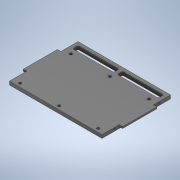
# Autodesk Inventor part: Cockpit_circuit_board_frame
Saved by Autodesk Inventor 2020.4 (Build 244396000, 396)
## iProperties
Created: 2022-01-28
Part Number: Cockpit_circuit_board_frame
Material: アセタール樹脂、黒
Document SubType Name: Modeling
Designer: Masato Kubotera
Density: 1.425 g/cm^3
Appearance: 滑らか - 黒
Author: Masato Kubotera
Autodesk Inventor part; units mm, degrees
ref_plane "YZ Plane" through (0, 0, 0) normal (1, 0, 0) x (0, 1, 0)
derived "Cockpit_side_frame.ipt"
sketch "スケッチ2" plane through (0, 0, 0) normal (0, 1, 0) x (-1, 0, 0)
  line L0 (-28.5, -22.5) -> (86.5, -22.5) construction
  line L1 (86.5, -22.5) -> (86.5, -138.5)
  line L2 (86.5, -96) -> (-28.5, -96) construction
  line L3 (-28.5, -96) -> (-28.5, -22.5) construction
  line L4 (-28.5, -22.5) -> (86.5, -96) construction
  line L5 (86.5, -22.5) -> (-28.5, -96) construction
  line L6 (36.5, -101) -> (36.5, -133.5)
  line L7 (41.5, -138.5) -> (86.5, -138.5)
  arc A0 (62.6349, -70.4) -> (61.15, -71.8849) centre (61.8925, -71.1425) ccw
  arc A1 (71.15, -72.5349) -> (69.6651, -71.05) centre (70.4075, -71.7925) ccw
  line L8 (63.3349, -71.05) -> (69.6651, -71.05)
  line L9 (62.6349, -70.4) -> (70.3651, -70.4)
  line L10 (61.9, -71.1) -> (71.1, -71.1) construction
  arc A2 (63.3349, -71.05) -> (61.85, -72.5349) centre (62.5925, -71.7925) ccw
  line L11 (61.2, -70.45) -> (71.8, -70.45) construction
  line L12 (71.15, -72.5349) -> (71.15, -83.4651)
  line L13 (71.8, -78) -> (61.2, -78) construction
  line L14 (71.85, -71.8849) -> (71.85, -84.1151)
  line L15 (71.1, -71.1) -> (71.1, -84.9) construction
  line L16 (61.85, -72.5349) -> (61.85, -83.4651)
  line L17 (71.8, -70.45) -> (71.8, -85.55) construction
  line L18 (61.15, -71.8849) -> (61.15, -84.1151)
  line L19 (66.5, -70.45) -> (66.5, -85.55) construction
  line L20 (61.9, -84.9) -> (61.9, -71.1) construction
  line L21 (71.1, -71.1) -> (61.9, -84.9) construction
  line L22 (71.8, -70.45) -> (61.2, -85.55) construction
  line L23 (61.2, -70.45) -> (71.8, -85.55) construction
  line L24 (61.2, -85.55) -> (61.2, -70.45) construction
  line L25 (61.9, -71.1) -> (71.1, -84.9) construction
  arc A3 (71.85, -71.8849) -> (70.3651, -70.4) centre (71.1075, -71.1425) ccw
  line L26 (71.1, -84.9) -> (61.9, -84.9) construction
  line L27 (71.8, -85.55) -> (61.2, -85.55) construction
  arc A4 (61.85, -83.4651) -> (63.3349, -84.95) centre (62.5925, -84.2075) ccw
  arc A5 (61.15, -84.1151) -> (62.6349, -85.6) centre (61.8925, -84.8575) ccw
  line L28 (63.3349, -84.95) -> (69.6651, -84.95)
  line L29 (62.6349, -85.6) -> (70.3651, -85.6)
  arc A6 (69.6651, -84.95) -> (71.15, -83.4651) centre (70.4075, -84.2075) ccw
  arc A7 (70.3651, -85.6) -> (71.85, -84.1151) centre (71.1075, -84.8575) ccw
  line L30 (-23.5, -22.5) -> (-28.5, -27.5)
  line L31 (-28.5, -59.25) -> (86.5, -59.25) construction
  line L32 (29, -22.5) -> (29, -96) construction
  line L33 (-23.5, -96) -> (-28.5, -91)
  line L34 (-28.5, -27.5) -> (-28.5, -91)
  line L35 (-21, -25) -> (-26, -25) construction
  line L36 (-26, -25) -> (-26, -93.5) construction
  line L37 (-26, -93.5) -> (-21, -93.5) construction
  line L38 (-21, -93.5) -> (-21, -25) construction
  line L39 (-21, -25) -> (-26, -93.5) construction
  line L40 (-26, -25) -> (-21, -93.5) construction
  line L41 (-26.05, -46.7) -> (-20.95, -46.7)
  line L42 (-20.95, -46.7) -> (-20.95, -71.8)
  line L43 (-20.95, -71.8) -> (-26.05, -71.8)
  line L44 (-26.05, -71.8) -> (-26.05, -46.7)
  line L45 (-26.05, -46.7) -> (-20.95, -71.8) construction
  line L46 (-20.95, -46.7) -> (-26.05, -71.8) construction
  line L47 (-26, -46.75) -> (-21, -46.75) construction
  line L48 (-26, -71.75) -> (-21, -71.75) construction
  line L49 (-23.5, -25) -> (-23.5, -93.5) construction
  circle A8 centre (-23.5, -35) radius 3
  circle A9 centre (-23.5, -35) radius 1.6
  arc A10 (-24.5651, -46.7) -> (-26.05, -48.1849) centre (-25.3075, -47.4425) ccw
  arc A11 (-20.95, -48.1849) -> (-22.4349, -46.7) centre (-21.6925, -47.4425) ccw
  arc A12 (-22.4349, -71.8) -> (-20.95, -70.3151) centre (-21.6925, -71.0575) ccw
  arc A13 (-26.05, -70.3151) -> (-24.5651, -71.8) centre (-25.3075, -71.0575) ccw
  circle A14 centre (-23.5, -83.5) radius 1.6
  circle A15 centre (-23.5, -83.5) radius 3
  line L50 (31.5, -96) -> (36.5, -101)
  line L51 (-23.5, -96) -> (31.5, -96)
  line L52 (79, -67.5) -> (-21, -67.5) construction
  line L53 (-21, -67.5) -> (-21, -62.5) construction
  line L54 (-21, -62.5) -> (79, -62.5) construction
  line L55 (79, -62.5) -> (79, -67.5) construction
  line L56 (79, -67.5) -> (-21, -62.5) construction
  line L57 (-21, -67.5) -> (79, -62.5) construction
  line L58 (-21, -65) -> (79, -65) construction
  line L59 (29, -62.5) -> (29, -67.5) construction
  line L60 (4, -62.5) -> (4, -67.5) construction
  line L61 (54.05, -62.45) -> (3.95, -62.45)
  line L62 (3.95, -62.45) -> (3.95, -67.55)
  line L63 (3.95, -67.55) -> (54.05, -67.55)
  line L64 (54.05, -67.55) -> (54.05, -62.45)
  line L65 (54.05, -62.45) -> (3.95, -67.55) construction
  line L66 (3.95, -62.45) -> (54.05, -67.55) construction
  arc A16 (5.4349, -62.45) -> (3.95, -63.9349) centre (4.6925, -63.1925) ccw
  circle A17 centre (-3.5, -65) radius 3
  circle A18 centre (-3.5, -65) radius 1.6
  line L67 (54, -62.5) -> (54, -67.5) construction
  arc A19 (54.05, -63.9349) -> (52.5651, -62.45) centre (53.3075, -63.1925) ccw
  circle A20 centre (61.5, -65) radius 3
  circle A21 centre (61.5, -65) radius 1.6
  arc A22 (3.95, -66.0651) -> (5.4349, -67.55) centre (4.6925, -66.8075) ccw
  arc A23 (52.5651, -67.55) -> (54.05, -66.0651) centre (53.3075, -66.8075) ccw
  line L68 (-21, -88.5) -> (79, -88.5) construction
  line L69 (79, -88.5) -> (79, -93.5) construction
  line L70 (79, -93.5) -> (-21, -93.5) construction
  line L71 (-21, -93.5) -> (-21, -88.5) construction
  line L72 (-21, -88.5) -> (79, -93.5) construction
  line L73 (79, -88.5) -> (-21, -93.5) construction
  line L74 (-21, -91) -> (79, -91) construction
  line L75 (29, -88.5) -> (29, -93.5) construction
  line L76 (54.05, -91.05) -> (3.95, -91.05)
  line L77 (3.95, -91.05) -> (3.95, -88.45)
  line L78 (3.95, -88.45) -> (54.05, -88.45)
  line L79 (54.05, -88.45) -> (54.05, -91.05)
  line L80 (54.05, -91.05) -> (3.95, -88.45) construction
  line L81 (3.95, -91.05) -> (54.05, -88.45) construction
  line L82 (4, -88.5) -> (4, -91) construction
  line L83 (54, -88.5) -> (54, -91) construction
  line L84 (4, -89.75) -> (54, -89.75) construction
  arc A24 (6.05, -88.45) -> (3.95, -88.45) centre (5, -88.45) ccw
  arc A25 (54.05, -88.45) -> (51.95, -88.45) centre (53, -88.45) ccw
  arc A26 (51.95, -91.05) -> (54.05, -91.05) centre (53, -91.05) ccw
  arc A27 (3.95, -91.05) -> (6.05, -91.05) centre (5, -91.05) ccw
  circle A28 centre (-3.5, -91) radius 3
  circle A29 centre (-3.5, -91) radius 1.6
  circle A30 centre (61.5, -91) radius 3 construction
  circle A31 centre (61.5, -91) radius 1.6 construction
  line L85 (-23.5, -22.5) -> (64.25, -22.5)
  line L86 (64.25, -22.5) -> (64.25, -17.5)
  line L87 (64.25, -17.5) -> (72.25, -17.5)
  line L88 (72.25, -17.5) -> (72.25, -22.5)
  line L89 (72.25, -22.5) -> (79, -22.5)
  line L90 (79, -22.5) -> (79, -17.5)
  line L91 (86.5, -22.5) -> (86.5, -20)
  line L92 (79, -17.5) -> (84, -17.5)
  line L93 (84, -17.5) -> (86.5, -20)
  line L94 (68.25, -17.5) -> (68.25, -22.5) construction
  arc A32 (62.7651, -22.5) -> (64.25, -21.0151) centre (63.5075, -21.7575) ccw
  arc A33 (72.25, -21.0151) -> (73.7349, -22.5) centre (72.9925, -21.7575) ccw
  arc A34 (77.5151, -22.5) -> (79, -21.0151) centre (78.2575, -21.7575) ccw
  line L95 (-16, -88.5) -> (-16, -68.5) construction
  line L96 (-16, -68.5) -> (64, -68.5) construction
  line L97 (64, -68.5) -> (64, -88.5) construction
  line L98 (45.5, -86) -> (-16.5, -86)
  line L99 (-18.5, -84) -> (-18.5, -72)
  line L100 (-16.5, -70) -> (45.5, -70)
  line L101 (47.5, -72) -> (47.5, -84)
  line L102 (47.5, -86) -> (-18.5, -70) construction
  line L103 (-18.5, -86) -> (47.5, -70) construction
  arc A35 (-16.5, -70) -> (-18.5, -72) centre (-16.5, -72) ccw
  arc A36 (-18.5, -84) -> (-16.5, -86) centre (-16.5, -84) ccw
  arc A37 (45.5, -86) -> (47.5, -84) centre (45.5, -84) ccw
  arc A38 (47.5, -72) -> (45.5, -70) centre (45.5, -72) ccw
  line L104 (36.5, -133.5) -> (41.5, -138.5)
  line L105 (44, -131) -> (39, -131) construction
  line L106 (39, -131) -> (39, -96) construction
  line L107 (39, -96) -> (44, -96) construction
  line L108 (44, -96) -> (44, -131) construction
  line L109 (44, -131) -> (39, -96) construction
  line L110 (39, -131) -> (44, -96) construction
  line L111 (41.5, -96) -> (41.5, -131) construction
  line L112 (39, -113.5) -> (44, -113.5) construction
  line L113 (41.5, -107.5) -> (44, -107.5) construction
  line L114 (41.45, -107.45) -> (44.05, -107.45)
  line L115 (44.05, -107.45) -> (44.05, -119.55)
  line L116 (44.05, -119.55) -> (41.45, -119.55)
  line L117 (41.45, -119.55) -> (41.45, -107.45)
  line L118 (41.45, -107.45) -> (44.05, -119.55) construction
  line L119 (44.05, -107.45) -> (41.45, -119.55) construction
  arc A39 (44.05, -109.55) -> (44.05, -107.45) centre (44.05, -108.5) ccw
  arc A40 (42.9349, -107.45) -> (41.45, -108.9349) centre (42.1925, -108.1925) ccw
  arc A41 (44.05, -119.55) -> (44.05, -117.45) centre (44.05, -118.5) ccw
  line L120 (41.5, -119.5) -> (44, -119.5) construction
  arc A42 (41.45, -118.0651) -> (42.9349, -119.55) centre (42.1925, -118.8075) ccw
  line L121 (42.75, -107.5) -> (42.75, -119.5) construction
  circle A43 centre (41.5, -125.5) radius 3 construction
  circle A44 centre (41.5, -125.5) radius 1.6 construction
  circle A45 centre (41.5, -101.5) radius 3
  circle A46 centre (41.5, -101.5) radius 1.6
  circle A47 centre (-13.5, -55) radius 2
  line L122 (39, -131) -> (77.8645, -131) construction
  line L123 (77.8645, -131) -> (77.8645, -136) construction
  line L124 (77.8645, -136) -> (39, -136) construction
  line L125 (39, -136) -> (39, -131) construction
  line L126 (39, -131) -> (77.8645, -136) construction
  line L127 (77.8645, -131) -> (39, -136) construction
  line L128 (39, -133.5) -> (77.8645, -133.5) construction
  line L129 (58.4322, -131) -> (58.4322, -136) construction
  line L130 (58.4322, -133.5) -> (58.4322, -131) construction
  line L131 (50.8822, -130.95) -> (65.9822, -130.95)
  line L132 (65.9822, -130.95) -> (65.9822, -133.55)
  line L133 (65.9822, -133.55) -> (50.8822, -133.55)
  line L134 (50.8822, -133.55) -> (50.8822, -130.95)
  line L135 (50.8822, -130.95) -> (65.9822, -133.55) construction
  line L136 (65.9822, -130.95) -> (50.8822, -133.55) construction
  line L137 (50.9322, -131) -> (50.9322, -133.5) construction
  arc A48 (52.9822, -130.95) -> (50.8822, -130.95) centre (51.9322, -130.95) ccw
  arc A49 (50.8822, -132.0651) -> (52.3672, -133.55) centre (51.6247, -132.8075) ccw
  arc A50 (65.9822, -130.95) -> (63.8822, -130.95) centre (64.9322, -130.95) ccw
  arc A51 (64.4973, -133.55) -> (65.9822, -132.0651) centre (65.2398, -132.8075) ccw
  line L138 (65.9322, -131) -> (65.9322, -133.5) construction
  line L139 (50.9322, -132.25) -> (65.9322, -132.25) construction
  circle A52 centre (72.4322, -133.5) radius 1.6 construction
  circle A53 centre (72.4322, -133.5) radius 3 construction
  circle A54 centre (44.4322, -133.5) radius 3
  circle A55 centre (44.4322, -133.5) radius 1.6
  line L140 (48.5, -96) -> (77, -96)
  line L141 (79, -98) -> (79, -126.5)
  line L142 (77, -128.5) -> (48.5, -128.5)
  line L143 (46.5, -126.5) -> (46.5, -98)
  line L144 (46.5, -96) -> (79, -128.5) construction
  line L145 (79, -96) -> (46.5, -128.5) construction
  arc A56 (48.5, -96) -> (46.5, -98) centre (48.5, -98) ccw
  arc A57 (46.5, -126.5) -> (48.5, -128.5) centre (48.5, -126.5) ccw
  arc A58 (77, -128.5) -> (79, -126.5) centre (77, -126.5) ccw
  arc A59 (79, -98) -> (77, -96) centre (77, -98) ccw
  line L146 (79, -91.1738) -> (84, -91.1738) construction
  line L147 (84, -91.1738) -> (84, -136) construction
  line L148 (84, -136) -> (79, -136) construction
  line L149 (79, -136) -> (79, -91.1738) construction
  line L150 (79, -91.1738) -> (84, -136) construction
  line L151 (84, -91.1738) -> (79, -136) construction
  line L152 (81.5, -91.1738) -> (81.5, -136) construction
  circle A60 centre (81.5, -93.6738) radius 1.475
  circle A61 centre (81.5, -98.6738) radius 1.475
  circle A62 centre (81.5, -103.6738) radius 1.475
  circle A63 centre (81.5, -133.5) radius 1.6
  arc A64 (84, -91.1738) -> (79, -91.1738) centre (81.5, -133.5) ccw construction
  arc A65 (84.0111, -91.0742) -> (78.9889, -91.0742) centre (81.5, -133.5) ccw construction
  line L153 (86.5, -133.5) -> (81.5, -138.5)
  arc A66 (79, -131) -> (84, -136) centre (81.5, -133.5) ccw construction
  line L154 (79, -65) -> (84, -65) construction
  line L155 (84, -65) -> (84, -91) construction
  line L156 (84, -91) -> (79, -91) construction
  line L157 (79, -91) -> (79, -65) construction
  line L158 (79, -65) -> (84, -91) construction
  line L159 (84, -65) -> (79, -91) construction
  line L160 (79, -78) -> (84, -78) construction
  line L161 (81.5, -65) -> (81.5, -91) construction
  line L162 (79, -73) -> (84, -73) construction
  line L163 (78.95, -72.95) -> (86.5, -72.95)
  line L164 (84.05, -72.95) -> (84.05, -83.05) construction
  line L165 (84.05, -83.05) -> (78.95, -83.05)
  line L166 (78.95, -83.05) -> (78.95, -72.95)
  line L167 (78.95, -72.95) -> (84.05, -83.05) construction
  line L168 (84.05, -72.95) -> (78.95, -83.05) construction
  arc A67 (80.4349, -72.95) -> (78.95, -74.4349) centre (79.6925, -73.6925) ccw
  arc A68 (78.95, -81.5651) -> (80.4349, -83.05) centre (79.6925, -82.3075) ccw
  line L169 (79, -83) -> (84, -83) construction
  circle A69 centre (81.5, -68) radius 1.6
  circle A70 centre (81.5, -68) radius 3
  circle A71 centre (81.5, -88) radius 1.6
  circle A72 centre (81.5, -88) radius 3
  line L170 (84.05, -83.05) -> (86.5, -83.05)
  circle A73 centre (81.5, -133.5) radius 3
  line L171 (75.625, -22.5) -> (75.625, -27.147) construction
  line L172 (60.875, -22.5) -> (60.875, -27.147) construction
  line L173 (64.25, -22.5) -> (72.25, -22.5)
  point P0 (0, 0)
  point P1 (29, -59.25)
  point P2 (-25.7227, -96)
  point P3 (61.85, -71.05)
  point P4 (61.15, -70.4)
  point P5 (66.5, -78)
  point P6 (-23.5, -59.25)
  point P7 (29, -65)
  point P8 (29, -91)
  point P9 (29, -89.75)
  point P10 (29, -89.75)
  point P11 (52.5, -22)
  point P12 (14.5, -78)
  point P13 (-18.5, -61)
  point P14 (47.5, -61)
  point P15 (41.5, -113.5)
  point P16 (42.75, -113.5)
  point P17 (58.4322, -133.5)
  point P18 (58.4322, -132.25)
  point P19 (62.75, -112.25)
  point P20 (81.5, -113.5869)
  point P21 (81.5, -78)
  dimension "d1" = 88.5
  dimension "d2" = 5
  dimension "d3" = 2.5
  measures "d1" vertical distance of L68.start point (0, 0)
  measures "d2" distance of L69.end L68.end
  measures "d3" distance of L83.start L83.end
ref_plane "作業平面1" through (0, 0, -88.5) normal (0, 0, 1) x (1, 0, 0)
sketch "スケッチ3" plane through (0, 0, -88.5) normal (0, 0, 1) x (1, 0, 0)
  line L0 (-79, -135) -> (21, -135)
  line L1 (21, -135) -> (21, 0)
  line L2 (21, 0) -> (-79, 0)
  line L3 (-79, 0) -> (-79, -135)
  line L4 (-79, -135) -> (21, 0) construction
  line L5 (21, -135) -> (-79, 0) construction
  line L6 (-4, 0) -> (-4, 5)
  line L7 (-4, 5) -> (-54, 5)
  line L8 (-54, 5) -> (-54, 0)
  arc A0 (-4, 1.4849) -> (-2.5151, 0) centre (-3.2575, 0.7425) ccw
  line L9 (-29, 0) -> (-29, -135) construction
  line L10 (21, -67.5) -> (-79, -67.5) construction
  arc A1 (-55.4849, 0) -> (-54, 1.4849) centre (-54.7425, 0.7425) ccw
  line L11 (-58, -124.5) -> (16, -124.5) construction
  line L12 (16, -124.5) -> (16, -10.5) construction
  line L13 (16, -10.5) -> (-58, -10.5) construction
  line L14 (-58, -10.5) -> (-58, -124.5) construction
  line L15 (-58, -124.5) -> (16, -10.5) construction
  line L16 (16, -124.5) -> (-58, -10.5) construction
  line L17 (-21, -10.5) -> (-21, -124.5) construction
  circle A2 centre (16, -10.5) radius 2
  circle A3 centre (-58, -10.5) radius 2
  line L18 (-45.8021, -123) -> (9.1979, -123) construction
  line L19 (9.1979, -123) -> (9.1979, -12) construction
  line L20 (9.1979, -12) -> (-45.8021, -12) construction
  line L21 (-45.8021, -12) -> (-45.8021, -123) construction
  line L22 (-45.8021, -123) -> (9.1979, -12) construction
  line L23 (9.1979, -123) -> (-45.8021, -12) construction
  circle A4 centre (16, -67.5) radius 2
  circle A5 centre (-58, -67.5) radius 2
  circle A6 centre (16, -124.5) radius 2
  circle A7 centre (-58, -124.5) radius 2
  line L24 (-68, -5) -> (-72, -5)
  line L25 (-74, -7) -> (-74, -63)
  line L26 (-72, -65) -> (-68, -65)
  line L27 (-66, -63) -> (-66, -7)
  line L28 (-66, -5) -> (-74, -65) construction
  line L29 (-74, -5) -> (-66, -65) construction
  line L30 (19, -7.5) -> (-61, -7.5) construction
  line L31 (-61, -7.5) -> (-61, -127.5) construction
  line L32 (-61, -127.5) -> (19, -127.5) construction
  line L33 (19, -127.5) -> (19, -7.5) construction
  line L34 (19, -7.5) -> (-61, -127.5) construction
  line L35 (-61, -7.5) -> (19, -127.5) construction
  arc A8 (-72, -5) -> (-74, -7) centre (-72, -7) ccw
  arc A9 (-74, -63) -> (-72, -65) centre (-72, -63) ccw
  arc A10 (-68, -65) -> (-66, -63) centre (-68, -63) ccw
  arc A11 (-66, -7) -> (-68, -5) centre (-68, -7) ccw
  line L36 (-68, -130) -> (-72, -130)
  line L37 (-74, -128) -> (-74, -72)
  line L38 (-66, -72) -> (-66, -128)
  arc A12 (-74, -128) -> (-72, -130) centre (-72, -128) ccw
  arc A13 (-72, -70) -> (-74, -72) centre (-72, -72) ccw
  arc A14 (-66, -72) -> (-68, -70) centre (-68, -72) ccw
  arc A15 (-68, -130) -> (-66, -128) centre (-68, -128) ccw
  line L39 (-72, -70) -> (-68, -70)
  line L40 (-4, -270) -> (-4, -275)
  line L41 (-4, -275) -> (-54, -275)
  line L42 (-54, -275) -> (-54, -270)
  arc A16 (-2.5151, -270) -> (-4, -271.4849) centre (-3.2575, -270.7425) ccw
  arc A17 (-54, -271.4849) -> (-55.4849, -270) centre (-54.7425, -270.7425) ccw
  line L43 (-4, -135) -> (-4, -140)
  line L44 (-4, -140) -> (-54, -140)
  line L45 (-54, -140) -> (-54, -135)
  arc A18 (-2.5151, -135) -> (-4, -136.4849) centre (-3.2575, -135.7425) ccw
  arc A19 (-54, -136.4849) -> (-55.4849, -135) centre (-54.7425, -135.7425) ccw
  point P0 (0, 0)
  point P1 (-29, -67.5)
  point P2 (-79, 0)
  point P3 (-54, 0)
  point P4 (-21, -67.5)
  point P5 (-18.3021, -67.5)
  point P6 (-60, -67.5)
  point P7 (-56, -67.5)
  point P8 (14, -67.5)
  point P9 (18, -67.5)
  point P10 (-54, 0)
  point P11 (-55.4849, 0)
  point P12 (-54, 1.4849)
  point P13 (-70, -35)
  point P14 (-54, -270)
  point P15 (-29, -270)
  point P16 (-54, -136.4849)
  point P17 (-55.4849, -135)
  point P18 (-2.5151, -135)
  dimension "d5" = 5
  dimension "d6" = 1.05
  dimension "d7" = 135
  dimension "d8" = 74
  dimension "d9" = 114
  dimension "d10" = 4
  dimension "d11" = 55
  dimension "d12" = 111
  dimension "d13" = 5
  dimension "d14" = 4
  dimension "d26" = 5
  dimension "d27" = 80
  dimension "d28" = 120
  dimension "d29" = 5
  dimension "d30" = 5
  dimension "d31" = 2.5
  dimension "d32" = 2
  constraints: 92 end point, 52 symmetric about line, 29 point on circle, 20 centre point, 17 midpoint, 16 point on line, 10 parallel, 9 coincident, 8 tangent, 7 perpendicular, 5 horizontal, 3 equal radius, 1 vertical, 13 other
  measures "d5" distance of L6.start L6.end
  measures "d6" radius of A0
  measures "d7" distance of L0.end L1.end
  measures "d8" distance of L13.end L12.end
  measures "d9" distance of L12.end L11.end
  measures "d10" diameter of A2
  measures "d11" distance of L20.end L19.end
  measures "d12" distance of L19.end L18.end
  measures "d13" horizontal distance of L12.end L1.end
  measures "d14" diameter of A4
  measures "d26" horizontal distance of L2.end L29.start
  measures "d27" distance of L32.end L31.end
  measures "d28" distance of L31.end L30.end
  measures "d29" horizontal distance of L2.end L29.start
  measures "d30" horizontal distance of L28.start L30.end
  measures "d31" vertical distance of L10.end L28.end
  measures "d32" radius of A8
extrude "押し出し1" add sketch "スケッチ3" against normal blind 5 contours L3 L2 A1 A0 L1 L0 A18 A19
extrude "押し出し2" add sketch "スケッチ3" against normal blind 2.5 contours L0 A18 L43 L44 L45 A19 | A1 L8 L7 L6 A0 L2
hole "穴1" at (3.5, 0, -91) at (-61.5, 0, -91) direction (0, -1, 0) diameter 3.242 depth 5 tip angle 118 thread size "M4x0.7" class "6H" standard "ISO Metric profile"
ref_plane "作業平面2" through (0, -67.5, 0) normal (0, 1, 0) x (-1, 0, 0)
mirror "ミラー1" about plane through (0, -67.5, 0) normal (0, 1, 0) of "穴1"
ref_plane "作業平面3" through (0, -67.5, 0) normal (0, 1, 0) x (-1, 0, 0)
equation "\"d14\" = d10"
equation "\"d29\" = d26"
equation "\"d30\" = d26"
equation "\"d31\" = 0.5 * d26"
equation "\"d15\" = d2"
equation "\"d17\" = d3"
equation "\"d4\" = -d1"
